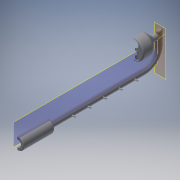
# Autodesk Inventor part: lampa_nadrazni
Saved by Autodesk Inventor 2018 (Build 220112000, 112)
## iProperties
Created: 2018-12-13
Part Number: lampa_nadrazni
Material: Generic
Document SubType Name: Modeling
Designer: petal
Density: 1 g/cm^3
Appearance: Default
Author: petal
Autodesk Inventor part; units mm, degrees
ref_plane "YZ Plane" through (0, 0, 0) normal (1, 0, 0) x (0, 1, 0)
ref_plane "XZ Plane" through (0, 0, 0) normal (0, 1, 0) x (-1, 0, 0)
ref_plane "XY Plane" through (0, 0, 0) normal (0, 0, 1) x (1, 0, 0)
sketch "Sketch1" plane through (0, 0, 0) normal (0, 0, 1) x (1, 0, 0)
  line L0 (0, 0) -> (0, 160)
  line L1 (0, 160) -> (4, 160) construction
  line L2 (4, 160) -> (4, 40)
  line L3 (0, 0) -> (8, 0)
  line L4 (8, 0) -> (8, 40)
  line L5 (8, 40) -> (4, 40)
  line L6 (4.125, 1.5) -> (4.5, 1.5)
  line L7 (4.5, 1.5) -> (4.5, 0)
  line L8 (4.125, 1.5) -> (4.125, 5.5)
  line L9 (4.125, 5.5) -> (6.5, 5.5)
  line L10 (6.5, 5.5) -> (6.5, 38.5)
  line L11 (6.5, 38.5) -> (2.5, 38.5)
  line L12 (2.5, 160) -> (4, 160)
  line L13 (4.125, 5.5) -> (4.125, 5.5)
  line L14 (4.125, 5.5) -> (6.5, 5.5)
  line L15 (2.5, 38.5) -> (2.5, 160)
  dimension "d0" = 160
  dimension "d3" = 8
  dimension "d4" = 40
  dimension "d20" = 1.5
  dimension "d22" = 1.5
  dimension "d26" = 1.5
  dimension "d27" = 4
  dimension "d29" = 9
  dimension "d73" = 8.25
  dimension "d74" = 8.25
  dimension "d75" = 0
  dimension "d78" = 5
  dimension "d79" = 1.5
  constraints: 32 end point, 6 perpendicular, 5 vertical, 4 point on line, 3 horizontal, 1 collinear, 1 parallel
  measures "d0" distance of L0.start L0.end
  measures "d3" distance of L0.start L3.end
  measures "d4" distance of L3.end L4.end
  measures "d20" distance between parallel lines of L4 L10
  measures "d22" distance between parallel lines of L5 L11
  measures "d26" distance from line of L3.end L6
  measures "d27" distance of L8.end L6.start
  measures "d29" diameter of L7 L0
  measures "d73" diameter of L8 L0
  measures "d74" diameter of L13 L0
  measures "d75" distance between parallel lines of L9 L14
  measures "d78" diameter of L15 L0
  measures "d79" distance between parallel lines of L15 L2
revolve "Revolution1" add sketch "Sketch1" angle 360 about axis through (0, 0, 0) along (0, 1, 0)
fillet "Fillet1" radius 2 1 edges at (-8, 40, 0)
fillet "Fillet2" radius 1 1 edges at (-8, 0, 0)
sketch "Sketch17" plane through (0, 160, 0) normal (0, 1, 0) x (1, 0, 0)
  circle A0 centre (0, 0) radius 2.5 projected
  circle A1 centre (0, 0) radius 4 projected
sketch "Sketch18" plane through (0, 0, 0) normal (1, 0, 0) x (0, 1, 0)
  line L0 (160, 2.5) -> (160, -2.5) projected
  arc A0 (160, 0) -> (180, 20) centre (160, 20) ccw
  line L1 (180, 20) -> (180, 35)
  point P0 (0, 0)
  dimension "d80" = 20
  dimension "d81" = 20
  dimension "d82" = 15
  constraints: 2 end point, 2 point on circle, 1 centre point, 1 midpoint, 1 vertical
  measures "d80" radius of A0
  measures "d81" distance from line of L1.end L0
  measures "d82" vertical distance of L1.end A0.centre
sweep "Sweep2" add profiles "Sketch17" path "Sketch18" path curves A0 L1
ref_plane "Work Plane6" through (0, 180, 30) normal (0, 0, 1) x (1, 0, 0)
sketch "Sketch19" plane through (0, 180, 30) normal (0, 0, 1) x (1, 0, 0)
  circle A0 centre (0, 0) radius 4 construction
  circle A1 centre (0, 0) radius 2.5 construction
  line L0 (-2.5, -20) -> (-2.5, 0) construction
  line L1 (-4, -9.8227) -> (-4, 0)
  line L2 (-4, -9.8227) -> (-13, -18.8227)
  line L3 (-13, -18.8227) -> (-13, -27.8227)
  line L4 (-2.5, 0) -> (-2.5, -10.4441)
  line L5 (-2.5, -10.4441) -> (-11.5, -19.4441)
  line L6 (-11.5, -19.4441) -> (-11.5, -27.8227)
  line L7 (-4, 0) -> (-2.5, 0)
  line L8 (-13, -27.8227) -> (-11.5, -27.8227)
  line L9 (0, 0) -> (0, -10.3281)
  point P0 (0, -180)
  dimension "d87" = 9.8227
  dimension "d88" = 9
  dimension "d89" = 9
  dimension "d90" = 9
  constraints: 18 end point, 3 vertical, 2 horizontal alignment, 1 horizontal, 1 parallel, 1 point on line, 3 other
  measures "d87" distance of L1.end L1.start
  measures "d88" horizontal distance of L2.end L1.start
  measures "d89" distance of L2.end L3.end
  measures "d90" horizontal distance of L2.end L1.start
revolve "Revolution4" add sketch "Sketch19" angle 360 about axis through (0, 180, 30) along (0, -1, 0)
sketch "Sketch20" plane through (0, 180, 35) normal (0, 0, 1) x (1, 0, 0)
  circle A0 centre (0, 0) radius 2.5 projected
  circle A1 centre (0, 0) radius 4 projected
  point P0 (0, -180)
extrude "Extrusion10" add sketch "Sketch20" along normal blind 2 contours A0 | A1
sketch "Sketch21" plane through (0, 152.1773, 30) normal (0, -1, 0) x (1, 0, 0)
  circle A0 centre (0, 0) radius 11.5 projected
  circle A1 centre (0, 0) radius 13 projected
  circle A2 centre (0, -5) radius 2.75
  circle A3 centre (0, 5) radius 4.5
  point P0 (0, -30)
  dimension "d94" = 5
  dimension "d95" = 5
  dimension "d96" = 5.5
  dimension "d97" = 9
  constraints: 2 centre point
  measures "d94" distance of A2.centre A0.centre
  measures "d95" distance of A0.centre A3.centre
  measures "d96" diameter of A2
  measures "d97" diameter of A3
extrude "Extrusion11" add sketch "Sketch21" along normal blind 2 contours A0 | A1
sketch "Sketch25" plane through (0, 150.1773, 30) normal (0, -1, 0) x (1, 0, 0)
  arc A0 (-2.5, 0) -> (2.5, 0) centre (0, 0) ccw construction
  circle A1 centre (0, 0) radius 11.5
  circle A2 centre (0, 5) radius 4.5 construction
  circle A3 centre (0, -5) radius 2.75 construction
  circle A4 centre (0, 0) radius 13 projected
  point P0 (0, -30)
  dimension "d122" = 1.5
  constraints: 1 centre point, 1 coincident
  measures "d122" radial gap between concentric circles of A4 A1
extrude "Extrusion15" add sketch "Sketch25" along normal blind 2
sketch "Sketch11" plane through (0, 0, 0) normal (1, 0, 0) x (0, 1, 0)
  line L0 (184.9406, 50.4926) -> (0, 50.4926)
  line L1 (0, 50.4926) -> (0, -25.116)
  line L2 (0, -25.116) -> (184.9406, -25.116)
  line L3 (184.9406, -25.116) -> (184.9406, 50.4926)
  point P0 (0, 0)
  constraints: 8 end point, 2 parallel, 1 horizontal, 1 perpendicular
extrude "Extrusion4" cut sketch "Sketch11" against normal blind 20
fillet "Fillet7" radius 5 2 edges at (4, 170.1773, 30) (13, 161.1773, 30)
fillet "Fillet7" radius 2 3 edges at (4, 180, 37) (2.8284, 177.1716, 27.1716) (2.8284, 177.1716, 32.8284)
fillet "Fillet7" radius 2 1 edges at (13, 148.1773, 30)
ref_plane "Work Plane7" through (0, 176, 20) normal (0, -1, 0) x (1, 0, 0)
sketch "Sketch22" plane through (0, 176, 20) normal (0, -1, 0) x (1, 0, 0)
  line L0 (0, 12.5) -> (0, 7.5) projected
  spline S0 degree 6 poles (0, 7.5) (0.1829, 7.5) (0.3643, 7.5161) (0.5414, 7.5477) (0.7116, 7.5935) (0.8725, 7.6515) (1.1368, 7.7699) (1.2457, 7.827) (1.3488, 7.889) (1.446, 7.9554) (1.5376, 8.0255) (1.7165, 8.1783) (1.803, 8.2616) (1.8834, 8.3485) (1.9578, 8.4385) (2.0264, 8.5314) (2.1561, 8.7288) (2.2165, 8.8336) (2.2705, 8.9413) (2.318, 9.0515) (2.3592, 9.1641) (2.4288, 9.3952) (2.4571, 9.5139) (2.4785, 9.6343) (2.4928, 9.7557) (2.5, 9.8778) (2.5, 10.1228) (2.4928, 10.2454) (2.4783, 10.3675) (2.4567, 10.4884) (2.4281, 10.6076) (2.3582, 10.8386) (2.3171, 10.9506) (2.2697, 11.0602) (2.2159, 11.1673) (2.1558, 11.2716) (2.0019, 11.506) (1.9033, 11.6337) (1.7935, 11.7557) (1.6718, 11.8712) (1.5377, 11.9791) (1.2858, 12.1477) (1.1742, 12.2132) (1.0558, 12.2732) (0.9308, 12.3268) (0.7994, 12.373) (0.5578, 12.4394) (0.45, 12.4632) (0.3394, 12.4815) (0.2269, 12.4938) (0.1134, 12.5) (0, 12.5) knots 0 0 0 0 0 0 0 0.114266 0.114266 0.114266 0.114266 0.114266 0.202092 0.202092 0.202092 0.202092 0.202092 0.296961 0.296961 0.296961 0.296961 0.296961 0.397704 0.397704 0.397704 0.397704 0.397704 0.4999 0.4999 0.4999 0.4999 0.4999 0.60258 0.60258 0.60258 0.60258 0.60258 0.702826 0.702826 0.702826 0.702826 0.702826 0.834847 0.834847 0.834847 0.834847 0.834847 0.928804 0.928804 0.928804 0.928804 0.928804 1 1 1 1 1 1 1 projected
  point P0 (0, -20)
  constraints: 1 vertical alignment
extrude "Extrusion12" cut sketch "Sketch22" against normal blind 4
sketch "Sketch23" plane through (0, 180, 35) normal (0, 0, -1) x (-1, 0, 0)
  line L0 (0, -2.5) -> (0, 2.5) projected
  arc A0 (0, 2.5) -> (0, -2.5) centre (0, 0) ccw projected
  point P0 (0, -180)
extrude "Extrusion13" cut sketch "Sketch23" along normal blind 10
fillet "Fillet8" radius 1 5 edges at (1.7678, 178.2322, 28.2322) (1.7678, 178.2322, 31.7678) (2.5, 169.5559, 30) (11.5, 160.5559, 30) (2.5, 180, 35)
ref_plane "Work Plane8" through (3, 0, 0) normal (-1, 0, 0) x (0, 0, 1)
sketch "Sketch24" plane through (3, 0, 0) normal (-1, 0, 0) x (0, 0, 1)
  line L0 (-2.5, 160) -> (-2.5, 38.5) construction
  line L1 (-2.5, 38.5) -> (2.5, 38.5) construction
  line L2 (2.5, 38.5) -> (2.5, 160) construction
  line L3 (-2.5, 160) -> (2.5, 160) construction
  line L4 (0, 160) -> (0, 38.5)
  circle A0 centre (0, 146) radius 0.9
  circle A1 centre (0, 126) radius 0.9
  circle A2 centre (0, 106) radius 0.9
  circle A3 centre (0, 86) radius 0.9
  circle A4 centre (0, 66) radius 0.9
  point P0 (0, 0)
  dimension "d109" = 1.8
  dimension "d110" = 14
  dimension "d113" = 20
  constraints: 5 centre point, 2 end point, 2 midpoint, 1 point on line, 1 vertical, 8 other
  measures "d109" diameter of A0
  measures "d110" distance from line of L3 A0.centre
  measures "d113" distance of A0.centre A1.centre
extrude "Extrusion14" add sketch "Sketch24" against normal blind 5
fillet "Fillet9" radius 0.5 5 edges at (8, 66, -0.9) (8, 86, -0.9) (8, 106, -0.9) (8, 126, -0.9) (8, 146, -0.9)
equation "\"d22\" = d20"
equation "\"d95\" = d94"
body "Solid1"
